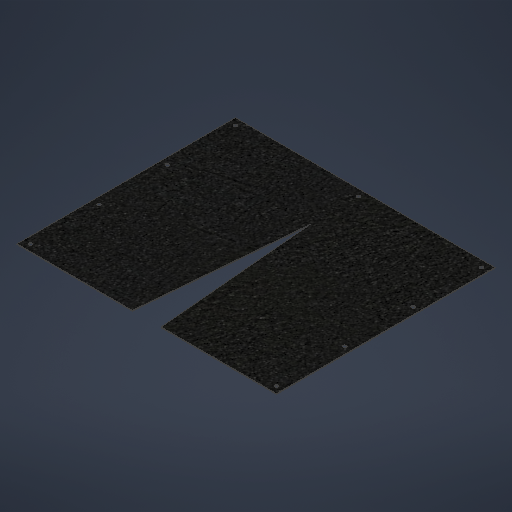
# Autodesk Inventor part: PuertaCuero
Saved by Autodesk Inventor 2026.2 (Build 302298010, 298A)
## iProperties
Created: 2026-04-15
Part Number: PuertaCuero
Material: Generic
Document SubType Name: Modeling
Designer: grego
Density: 1 g/cm^3
Appearance: Default
Author: grego
Autodesk Inventor part; units mm, degrees
ref_plane "YZ Plane" through (0, 0, 0) normal (1, 0, 0) x (0, 1, 0)
ref_plane "XZ Plane" through (0, 0, 0) normal (0, 1, 0) x (-1, 0, 0)
ref_plane "XY Plane" through (0, 0, 0) normal (0, 0, 1) x (1, 0, 0)
sketch "Sketch1" plane through (0, 0, 0) normal (0, 1, 0) x (-1, 0, 0)
  line L0 (190, 160) -> (-190, 160)
  line L1 (-190, 160) -> (-190, -160)
  line L2 (-190, -160) -> (190, -160)
  line L3 (190, -160) -> (190, 160)
  line L4 (0, -80) -> (20.9973, 160)
  line L5 (0, -80) -> (240.9168, -80) construction
  line L6 (0, -80) -> (-20.9973, 160)
  line L7 (180, -150) -> (-180, -150)
  line L8 (-180, -150) -> (-180, 150)
  line L9 (180, 150) -> (180, -150)
  circle A0 centre (180, 150) radius 2.5
  circle A1 centre (-180, 150) radius 2.5
  line L10 (180, 160) -> (180, 50)
  line L11 (180, 50) -> (180, -50)
  circle A2 centre (180, 50) radius 2.5
  circle A3 centre (180, -50) radius 2.5
  circle A4 centre (180, -150) radius 2.5
  circle A5 centre (-180, 50) radius 2.5
  circle A6 centre (-180, -50) radius 2.5
  circle A7 centre (-180, -150) radius 2.5
  circle A8 centre (0, -150) radius 2.5
  point P0 (0, 0)
  dimension "d0" = 380
  dimension "d1" = 320
  dimension "d2" = 85
  dimension "d3" = 10
  dimension "d4" = 5
  dimension "d5" = 5
  dimension "d6" = 110
  dimension "d7" = 100
  dimension "d8" = 5
  dimension "d9" = 5
  dimension "d10" = 5
  dimension "d11" = 5
  constraints: 24 end point, 9 centre point, 5 coincident, 4 point on line, 3 parallel, 2 horizontal, 1 equal length, 1 midpoint, 1 perpendicular, 1 other
  measures "d0" distance of L2.end L1.end
  measures "d1" distance of L1.end L0.end
  measures "d2" angle of L5 L4
  measures "d3" distance between parallel lines of L2 L7
  measures "d4" diameter of A0
  measures "d5" diameter of A1
  measures "d6" distance of L10.start L10.end
  measures "d7" distance of L10.end L11.end
  measures "d8" diameter of A2
  measures "d9" diameter of A3
  measures "d10" diameter of A4
  measures "d11" diameter of A8
extrude "Extrusion1" add sketch "Sketch1" along normal blind 1 contours L3 L2 L1 L0 L6 L4
body "Solid1"
